Autodesk Fusion 360 part; units mm, degrees
(part 2 of 2)
  spline S15 degree 5 poles (15.988634, 0.602981) (15.980531, 0.608149) (15.964319, 0.618461) (15.939982, 0.633849) (15.907494, 0.654209) (15.866821, 0.679398) (15.826084, 0.704324) (15.785284, 0.728987) (15.744422, 0.753386) (15.703497, 0.777518) (15.662512, 0.801383) (15.621467, 0.824978) (15.580364, 0.848302) (15.539203, 0.871354) (15.497987, 0.89413) (15.456715, 0.916631) (15.415389, 0.938854) (15.37401, 0.960797) (15.332579, 0.98246) (15.291097, 1.003839) (15.249564, 1.024933) (15.207982, 1.04574) (15.166352, 1.066257) (15.124674, 1.086484) (15.082952, 1.106417) (15.041184, 1.126055) (14.999373, 1.145396) (14.957519, 1.164437) (14.915624, 1.183176) (14.873688, 1.201611) (14.831714, 1.219738) (14.789702, 1.237554) (14.747652, 1.255057) (14.705568, 1.272243) (14.663449, 1.28911) (14.621297, 1.305656) (14.579113, 1.321879) (14.536899, 1.337776) (14.494656, 1.353344) (14.452384, 1.368578) (14.410087, 1.383471) (14.367764, 1.398017) (14.325417, 1.412211) (14.283049, 1.426048) (14.24066, 1.439527) (14.198251, 1.452649) (14.155825, 1.465414) (14.113381, 1.47782) (14.070923, 1.48986) (14.028452, 1.501522) (13.98597, 1.512783) (13.94348, 1.523626) (13.900982, 1.534034) (13.858481, 1.544002) (13.815976, 1.553541) (13.773469, 1.562672) (13.73096, 1.571415) (13.688453, 1.579774) (13.64595, 1.587728) (13.603455, 1.595217) (13.560973, 1.60215) (13.518509, 1.608443) (13.476069, 1.614042) (13.433654, 1.618949) (13.391265, 1.62326) (13.348902, 1.627116) (13.306566, 1.630627) (13.264262, 1.633807) (13.222004, 1.636509) (13.179816, 1.638338) (13.137727, 1.638758) (13.104158, 1.637534) (13.079047, 1.635547) (13.062338, 1.633722) (13.053992, 1.632684) knots -1 -1 -1 -1 -1 -1 -0.98571429 -0.97142857 -0.95714286 -0.94285714 -0.92857143 -0.91428571 -0.9 -0.88571429 -0.87142857 -0.85714286 -0.84285714 -0.82857143 -0.81428571 -0.8 -0.78571429 -0.77142857 -0.75714286 -0.74285714 -0.72857143 -0.71428571 -0.7 -0.68571429 -0.67142857 -0.65714286 -0.64285714 -0.62857143 -0.61428571 -0.6 -0.58571429 -0.57142857 -0.55714286 -0.54285714 -0.52857143 -0.51428571 -0.5 -0.48571429 -0.47142857 -0.45714286 -0.44285714 -0.42857143 -0.41428571 -0.4 -0.38571429 -0.37142857 -0.35714286 -0.34285714 -0.32857143 -0.31428571 -0.3 -0.28571429 -0.27142857 -0.25714286 -0.24285714 -0.22857143 -0.21428571 -0.2 -0.18571429 -0.17142857 -0.15714286 -0.14285714 -0.12857143 -0.11428571 -0.1 -0.08571429 -0.07142857 -0.05714286 -0.04285714 -0.02857143 -0.01428571 0 0 0 0 0 0
  line L15 (13.053992, 1.632684) -> (12.411729, 1.552852)
  arc A31 (11.309164, 2.342397) -> (12.411729, 1.552852) centre (12.288381, 2.545216) ccw
  arc A32 (11.309164, 2.342397) -> (11.205533, 2.796436) centre (0, 0) ccw
  arc A33 (11.856339, 3.986176) -> (11.205533, 2.796436) centre (12.175776, 3.038568) ccw
  line L16 (11.856339, 3.986176) -> (12.469635, 4.192917)
  spline S16 degree 5 poles (12.469635, 4.192917) (12.477606, 4.195604) (12.493452, 4.201209) (12.516938, 4.210313) (12.547714, 4.223776) (12.585452, 4.242417) (12.622669, 4.262369) (12.659569, 4.283138) (12.696304, 4.304359) (12.732924, 4.325891) (12.769419, 4.347745) (12.80574, 4.370021) (12.841825, 4.392845) (12.877633, 4.416304) (12.913161, 4.440398) (12.948428, 4.465077) (12.983466, 4.490262) (13.018309, 4.51587) (13.052979, 4.541844) (13.087484, 4.568165) (13.12182, 4.594835) (13.155977, 4.621871) (13.189945, 4.649293) (13.223717, 4.67711) (13.257296, 4.705314) (13.290684, 4.733893) (13.32389, 4.762827) (13.356919, 4.792097) (13.389776, 4.82169) (13.422463, 4.851599) (13.454978, 4.881822) (13.487322, 4.912358) (13.519491, 4.943207) (13.551485, 4.974369) (13.583305, 5.005838) (13.614952, 5.037608) (13.646428, 5.069674) (13.677733, 5.102029) (13.708869, 5.134668) (13.739836, 5.167588) (13.770635, 5.200784) (13.801264, 5.234256) (13.831724, 5.268) (13.862015, 5.302013) (13.892137, 5.336294) (13.92209, 5.370838) (13.951874, 5.405642) (13.981489, 5.440703) (14.010937, 5.476018) (14.040216, 5.511585) (14.069326, 5.5474) (14.098269, 5.583462) (14.127042, 5.619769) (14.155647, 5.656317) (14.184084, 5.693105) (14.212351, 5.730131) (14.24045, 5.767391) (14.268379, 5.804885) (14.296139, 5.842609) (14.32373, 5.880561) (14.351152, 5.918741) (14.378404, 5.957145) (14.405487, 5.995773) (14.4324, 6.034621) (14.459143, 6.073689) (14.485715, 6.112973) (14.512116, 6.152472) (14.538345, 6.192183) (14.564404, 6.232106) (14.590291, 6.272239) (14.616007, 6.312581) (14.636444, 6.345021) (14.651694, 6.369445) (14.661827, 6.385769) (14.666885, 6.393941) knots 0 0 0 0 0 0 0.01428571 0.02857143 0.04285714 0.05714286 0.07142857 0.08571429 0.1 0.11428571 0.12857143 0.14285714 0.15714286 0.17142857 0.18571429 0.2 0.21428571 0.22857143 0.24285714 0.25714286 0.27142857 0.28571429 0.3 0.31428571 0.32857143 0.34285714 0.35714286 0.37142857 0.38571429 0.4 0.41428571 0.42857143 0.44285714 0.45714286 0.47142857 0.48571429 0.5 0.51428571 0.52857143 0.54285714 0.55714286 0.57142857 0.58571429 0.6 0.61428571 0.62857143 0.64285714 0.65714286 0.67142857 0.68571429 0.7 0.71428571 0.72857143 0.74285714 0.75714286 0.77142857 0.78571429 0.8 0.81428571 0.82857143 0.84285714 0.85714286 0.87142857 0.88571429 0.9 0.91428571 0.92857143 0.94285714 0.95714286 0.97142857 0.98571429 1 1 1 1 1 1
  arc A34 (14.666885, 6.393941) -> (14.143638, 7.480475) centre (0, 0) ccw
  spline S17 degree 5 poles (14.143638, 7.480475) (14.134095, 7.481616) (14.115014, 7.483872) (14.086411, 7.487177) (14.048306, 7.491425) (14.000732, 7.496472) (13.953214, 7.501255) (13.905754, 7.505773) (13.858352, 7.510026) (13.81101, 7.514012) (13.763729, 7.51773) (13.716511, 7.52118) (13.669358, 7.52436) (13.622272, 7.52727) (13.575255, 7.529908) (13.528308, 7.532273) (13.481432, 7.534365) (13.43463, 7.536182) (13.387903, 7.537722) (13.341253, 7.538986) (13.29468, 7.53997) (13.248189, 7.540675) (13.201779, 7.541098) (13.155453, 7.541238) (13.109213, 7.541095) (13.063062, 7.540666) (13.016999, 7.53995) (12.971029, 7.538946) (12.925152, 7.537652) (12.879371, 7.536066) (12.833688, 7.534185) (12.788106, 7.532009) (12.742627, 7.529533) (12.697253, 7.526758) (12.651987, 7.52368) (12.606831, 7.520298) (12.561786, 7.516612) (12.516854, 7.512619) (12.472039, 7.508317) (12.427345, 7.503701) (12.382774, 7.498767) (12.338331, 7.493509) (12.29402, 7.487924) (12.249843, 7.482008) (12.205804, 7.47576) (12.161902, 7.469182) (12.118138, 7.462274) (12.074515, 7.455036) (12.031038, 7.447463) (11.987713, 7.439541) (11.944552, 7.431256) (11.901565, 7.422589) (11.85876, 7.413527) (11.816142, 7.404067) (11.773708, 7.394219) (11.731448, 7.384003) (11.689356, 7.373437) (11.647432, 7.362524) (11.605687, 7.35125) (11.564151, 7.339558) (11.522868, 7.327373) (11.481879, 7.314618) (11.441212, 7.301249) (11.400868, 7.287267) (11.360807, 7.272759) (11.320966, 7.257852) (11.281299, 7.242646) (11.241805, 7.227157) (11.20256, 7.211256) (11.163756, 7.194599) (11.125653, 7.176716) (11.095939, 7.161048) (11.074177, 7.148363) (11.059915, 7.139469) (11.052845, 7.134912) knots -1 -1 -1 -1 -1 -1 -0.98571429 -0.97142857 -0.95714286 -0.94285714 -0.92857143 -0.91428571 -0.9 -0.88571429 -0.87142857 -0.85714286 -0.84285714 -0.82857143 -0.81428571 -0.8 -0.78571429 -0.77142857 -0.75714286 -0.74285714 -0.72857143 -0.71428571 -0.7 -0.68571429 -0.67142857 -0.65714286 -0.64285714 -0.62857143 -0.61428571 -0.6 -0.58571429 -0.57142857 -0.55714286 -0.54285714 -0.52857143 -0.51428571 -0.5 -0.48571429 -0.47142857 -0.45714286 -0.44285714 -0.42857143 -0.41428571 -0.4 -0.38571429 -0.37142857 -0.35714286 -0.34285714 -0.32857143 -0.31428571 -0.3 -0.28571429 -0.27142857 -0.25714286 -0.24285714 -0.22857143 -0.21428571 -0.2 -0.18571429 -0.17142857 -0.15714286 -0.14285714 -0.12857143 -0.11428571 -0.1 -0.08571429 -0.07142857 -0.05714286 -0.04285714 -0.02857143 -0.01428571 0 0 0 0 0 0
  line L17 (11.052845, 7.134912) -> (10.508824, 6.784319)
  arc A35 (9.172877, 7.017289) -> (10.508824, 6.784319) centre (9.967121, 7.624889) ccw
  arc A36 (9.172877, 7.017289) -> (8.882508, 7.3814) centre (0, 0) ccw
  arc A37 (8.952656, 8.735693) -> (8.882508, 7.3814) centre (9.65161, 8.020527) ccw
  line L18 (8.952656, 8.735693) -> (9.415515, 9.18806)
  spline S18 degree 5 poles (9.415515, 9.18806) (9.42153, 9.193938) (9.433375, 9.205864) (9.450585, 9.224257) (9.472472, 9.24974) (9.498385, 9.282909) (9.523259, 9.317033) (9.547494, 9.351755) (9.571383, 9.386813) (9.595034, 9.422102) (9.618433, 9.457627) (9.641492, 9.493455) (9.6641, 9.529676) (9.686184, 9.566348) (9.707739, 9.603471) (9.728806, 9.641008) (9.749447, 9.678901) (9.769728, 9.717091) (9.789696, 9.755536) (9.809364, 9.794221) (9.828727, 9.833148) (9.847771, 9.872327) (9.866477, 9.911771) (9.884836, 9.951486) (9.902851, 9.991467) (9.920534, 10.031702) (9.937897, 10.072178) (9.954955, 10.11288) (9.971719, 10.153799) (9.988191, 10.194928) (10.004374, 10.236266) (10.020265, 10.277811) (10.035863, 10.319563) (10.051168, 10.36152) (10.066183, 10.403679) (10.080912, 10.446035) (10.095357, 10.488582) (10.109524, 10.531315) (10.123415, 10.574232) (10.137032, 10.617327) (10.150377, 10.660599) (10.163451, 10.704046) (10.176254, 10.747664) (10.188787, 10.791452) (10.201052, 10.835407) (10.21305, 10.879526) (10.224784, 10.923806) (10.236254, 10.968245) (10.247462, 11.012839) (10.25841, 11.057587) (10.269098, 11.102487) (10.279528, 11.147535) (10.289699, 11.19273) (10.299614, 11.238071) (10.309272, 11.283554) (10.318675, 11.329178) (10.327825, 11.37494) (10.33672, 11.420838) (10.345364, 11.466871) (10.353755, 11.513036) (10.361896, 11.559333) (10.369786, 11.605758) (10.377427, 11.652311) (10.384819, 11.698989) (10.391963, 11.745791) (10.398858, 11.792714) (10.405507, 11.839756) (10.411909, 11.886916) (10.418065, 11.934192) (10.423976, 11.981582) (10.429642, 12.029087) (10.433979, 12.067181) (10.437122, 12.095803) (10.439169, 12.114907) (10.44018, 12.124465) knots 0 0 0 0 0 0 0.01428571 0.02857143 0.04285714 0.05714286 0.07142857 0.08571429 0.1 0.11428571 0.12857143 0.14285714 0.15714286 0.17142857 0.18571429 0.2 0.21428571 0.22857143 0.24285714 0.25714286 0.27142857 0.28571429 0.3 0.31428571 0.32857143 0.34285714 0.35714286 0.37142857 0.38571429 0.4 0.41428571 0.42857143 0.44285714 0.45714286 0.47142857 0.48571429 0.5 0.51428571 0.52857143 0.54285714 0.55714286 0.57142857 0.58571429 0.6 0.61428571 0.62857143 0.64285714 0.65714286 0.67142857 0.68571429 0.7 0.71428571 0.72857143 0.74285714 0.75714286 0.77142857 0.78571429 0.8 0.81428571 0.82857143 0.84285714 0.85714286 0.87142857 0.88571429 0.9 0.91428571 0.92857143 0.94285714 0.95714286 0.97142857 0.98571429 1 1 1 1 1 1
  arc A38 (10.44018, 12.124465) -> (9.497321, 12.87637) centre (0, 0) ccw
  spline S19 degree 5 poles (9.497321, 12.87637) (9.488228, 12.873257) (9.470058, 12.867011) (9.442853, 12.857578) (9.406679, 12.844872) (9.361626, 12.828778) (9.316739, 12.81247) (9.272018, 12.795948) (9.227466, 12.779213) (9.183082, 12.762263) (9.13887, 12.745099) (9.094832, 12.72772) (9.050969, 12.710127) (9.007283, 12.692318) (8.963777, 12.674295) (8.920453, 12.656057) (8.877312, 12.637603) (8.834357, 12.618933) (8.791589, 12.600047) (8.74901, 12.580944) (8.706623, 12.561624) (8.664429, 12.542087) (8.622432, 12.522332) (8.580633, 12.502358) (8.539035, 12.482166) (8.49764, 12.461755) (8.45645, 12.441124) (8.415467, 12.420274) (8.374695, 12.399203) (8.334136, 12.37791) (8.293793, 12.356395) (8.253669, 12.334657) (8.213768, 12.312694) (8.174092, 12.290506) (8.134644, 12.268093) (8.095427, 12.245454) (8.056442, 12.222588) (8.017693, 12.199495) (7.979183, 12.176175) (7.940917, 12.152624) (7.902901, 12.12884) (7.86514, 12.10482) (7.827641, 12.080562) (7.790406, 12.056064) (7.753439, 12.031327) (7.716738, 12.006351) (7.680306, 11.98114) (7.644143, 11.955691) (7.608257, 11.930004) (7.57266, 11.904069) (7.537368, 11.877877) (7.502399, 11.851416) (7.467765, 11.82468) (7.433472, 11.797666) (7.399512, 11.770382) (7.365871, 11.742842) (7.332532, 11.715058) (7.299494, 11.687037) (7.266775, 11.658766) (7.234425, 11.630211) (7.202517, 11.60132) (7.171121, 11.572044) (7.140282, 11.542354) (7.110001, 11.512252) (7.080201, 11.481799) (7.050774, 11.451082) (7.021633, 11.420171) (6.99277, 11.38908) (6.964311, 11.357726) (6.936577, 11.325882) (6.910006, 11.293238) (6.890033, 11.266229) (6.875931, 11.245358) (6.86694, 11.231156) (6.862547, 11.223984) knots -1 -1 -1 -1 -1 -1 -0.98571429 -0.97142857 -0.95714286 -0.94285714 -0.92857143 -0.91428571 -0.9 -0.88571429 -0.87142857 -0.85714286 -0.84285714 -0.82857143 -0.81428571 -0.8 -0.78571429 -0.77142857 -0.75714286 -0.74285714 -0.72857143 -0.71428571 -0.7 -0.68571429 -0.67142857 -0.65714286 -0.64285714 -0.62857143 -0.61428571 -0.6 -0.58571429 -0.57142857 -0.55714286 -0.54285714 -0.52857143 -0.51428571 -0.5 -0.48571429 -0.47142857 -0.45714286 -0.44285714 -0.42857143 -0.41428571 -0.4 -0.38571429 -0.37142857 -0.35714286 -0.34285714 -0.32857143 -0.31428571 -0.3 -0.28571429 -0.27142857 -0.25714286 -0.24285714 -0.22857143 -0.21428571 -0.2 -0.18571429 -0.17142857 -0.15714286 -0.14285714 -0.12857143 -0.11428571 -0.1 -0.08571429 -0.07142857 -0.05714286 -0.04285714 -0.02857143 -0.01428571 0 0 0 0 0 0
  line L19 (6.862547, 11.223984) -> (6.524518, 10.672068)
  arc A39 (5.219789, 10.302321) -> (6.524518, 10.672068) centre (5.67175, 11.194359) ccw
  arc A40 (5.219789, 10.302321) -> (4.800194, 10.504388) centre (0, 0) ccw
  arc A41 (4.275789, 11.754999) -> (4.800194, 10.504388) centre (5.215824, 11.413921) ccw
  line L20 (4.275789, 11.754999) -> (4.496536, 12.363394)
  spline S20 degree 5 poles (4.496536, 12.363394) (4.499405, 12.371301) (4.504902, 12.387185) (4.512427, 12.411223) (4.52109, 12.443679) (4.530046, 12.484806) (4.537651, 12.526344) (4.54442, 12.568143) (4.550733, 12.610094) (4.556731, 12.65215) (4.562399, 12.694309) (4.567628, 12.736594) (4.572282, 12.779037) (4.576267, 12.82166) (4.579581, 12.864459) (4.582275, 12.907419) (4.58443, 12.950515) (4.586133, 12.993723) (4.587443, 13.037024) (4.588378, 13.080412) (4.588935, 13.123885) (4.589093, 13.167447) (4.588832, 13.211101) (4.588141, 13.254849) (4.587026, 13.298687) (4.5855, 13.34261) (4.583582, 13.386611) (4.581291, 13.430684) (4.57864, 13.474823) (4.575636, 13.519027) (4.57228, 13.563292) (4.568571, 13.607618) (4.564509, 13.652003) (4.560094, 13.696446) (4.555331, 13.740944) (4.550223, 13.785496) (4.544778, 13.830097) (4.539, 13.874746) (4.532895, 13.919439) (4.526465, 13.964175) (4.519713, 14.008952) (4.512641, 14.053768) (4.505251, 14.098622) (4.497544, 14.143511) (4.489523, 14.188435) (4.481191, 14.23339) (4.47255, 14.278377) (4.463603, 14.323391) (4.454353, 14.368433) (4.444801, 14.413499) (4.434949, 14.45859) (4.4248, 14.503702) (4.414355, 14.548835) (4.403615, 14.593987) (4.392583, 14.639156) (4.381259, 14.684342) (4.369647, 14.729542) (4.357747, 14.774754) (4.345562, 14.819979) (4.333092, 14.865213) (4.320339, 14.910457) (4.307305, 14.955709) (4.293991, 15.000966) (4.280397, 15.046229) (4.266527, 15.091496) (4.252381, 15.136764) (4.23796, 15.182032) (4.223266, 15.227299) (4.208301, 15.272564) (4.193064, 15.317826) (4.177557, 15.363084) (4.164936, 15.399288) (4.15535, 15.42644) (4.148905, 15.44454) (4.145669, 15.45359) knots 0 0 0 0 0 0 0.01428571 0.02857143 0.04285714 0.05714286 0.07142857 0.08571429 0.1 0.11428571 0.12857143 0.14285714 0.15714286 0.17142857 0.18571429 0.2 0.21428571 0.22857143 0.24285714 0.25714286 0.27142857 0.28571429 0.3 0.31428571 0.32857143 0.34285714 0.35714286 0.37142857 0.38571429 0.4 0.41428571 0.42857143 0.44285714 0.45714286 0.47142857 0.48571429 0.5 0.51428571 0.52857143 0.54285714 0.55714286 0.57142857 0.58571429 0.6 0.61428571 0.62857143 0.64285714 0.65714286 0.67142857 0.68571429 0.7 0.71428571 0.72857143 0.74285714 0.75714286 0.77142857 0.78571429 0.8 0.81428571 0.82857143 0.84285714 0.85714286 0.87142857 0.88571429 0.9 0.91428571 0.92857143 0.94285714 0.95714286 0.97142857 0.98571429 1 1 1 1 1 1
  arc A42 (4.145669, 15.45359) -> (2.969943, 15.721941) centre (0, 0) ccw
  spline S21 degree 5 poles (2.969943, 15.721941) (2.963101, 15.715192) (2.949441, 15.70168) (2.929023, 15.681378) (2.901944, 15.654235) (2.868336, 15.620187) (2.834969, 15.586018) (2.801846, 15.551729) (2.768967, 15.51732) (2.736333, 15.482792) (2.703947, 15.448144) (2.671809, 15.413379) (2.639924, 15.378496) (2.608291, 15.343497) (2.576914, 15.308383) (2.545793, 15.273153) (2.514932, 15.237808) (2.484331, 15.202349) (2.453993, 15.166777) (2.423919, 15.131092) (2.394112, 15.095294) (2.364574, 15.059385) (2.335307, 15.023364) (2.306313, 14.987233) (2.277596, 14.950992) (2.249156, 14.914641) (2.220996, 14.878182) (2.193119, 14.841614) (2.165527, 14.80494) (2.138223, 14.768158) (2.11121, 14.731269) (2.084492, 14.694274) (2.058072, 14.657174) (2.031952, 14.619969) (2.006135, 14.58266) (1.980624, 14.545246) (1.955421, 14.50773) (1.930529, 14.470112) (1.905951, 14.432392) (1.881693, 14.39457) (1.857761, 14.356647) (1.834162, 14.318622) (1.810901, 14.280496) (1.787983, 14.242269) (1.76541, 14.203942) (1.74318, 14.165516) (1.721295, 14.126994) (1.699755, 14.088375) (1.678568, 14.049661) (1.657749, 14.01085) (1.637316, 13.971939) (1.617291, 13.932926) (1.597687, 13.893811) (1.578511, 13.854593) (1.559753, 13.815276) (1.541392, 13.775866) (1.52341, 13.736369) (1.505802, 13.696788) (1.488589, 13.657121) (1.471832, 13.617357) (1.45562, 13.577483) (1.440035, 13.537484) (1.425133, 13.497354) (1.41091, 13.457094) (1.397275, 13.416728) (1.38409, 13.376284) (1.371246, 13.335791) (1.358732, 13.295256) (1.346694, 13.254659) (1.335524, 13.213935) (1.325748, 13.172995) (1.319471, 13.139995) (1.315822, 13.115072) (1.313883, 13.098376) (1.313037, 13.090007) knots -1 -1 -1 -1 -1 -1 -0.98571429 -0.97142857 -0.95714286 -0.94285714 -0.92857143 -0.91428571 -0.9 -0.88571429 -0.87142857 -0.85714286 -0.84285714 -0.82857143 -0.81428571 -0.8 -0.78571429 -0.77142857 -0.75714286 -0.74285714 -0.72857143 -0.71428571 -0.7 -0.68571429 -0.67142857 -0.65714286 -0.64285714 -0.62857143 -0.61428571 -0.6 -0.58571429 -0.57142857 -0.55714286 -0.54285714 -0.52857143 -0.51428571 -0.5 -0.48571429 -0.47142857 -0.45714286 -0.44285714 -0.42857143 -0.41428571 -0.4 -0.38571429 -0.37142857 -0.35714286 -0.34285714 -0.32857143 -0.31428571 -0.3 -0.28571429 -0.27142857 -0.25714286 -0.24285714 -0.22857143 -0.21428571 -0.2 -0.18571429 -0.17142857 -0.15714286 -0.14285714 -0.12857143 -0.11428571 -0.1 -0.08571429 -0.07142857 -0.05714286 -0.04285714 -0.02857143 -0.01428571 0 0 0 0 0 0
  line L21 (1.313037, 13.090007) -> (1.24795, 12.446084)
  arc A43 (0.232858, 11.546852) -> (1.24795, 12.446084) centre (0.25302, 12.546649) ccw
  arc A44 (0.232858, 11.546852) -> (-0.232858, 11.546852) centre (0, 0) ccw
  arc A45 (-1.24795, 12.446084) -> (-0.232858, 11.546852) centre (-0.25302, 12.546649) ccw
  line L22 (-1.24795, 12.446084) -> (-1.313037, 13.090007)
  spline S22 degree 5 poles (-1.313037, 13.090007) (-1.313883, 13.098376) (-1.315822, 13.115072) (-1.319471, 13.139995) (-1.325748, 13.172995) (-1.335524, 13.213935) (-1.346694, 13.254659) (-1.358732, 13.295256) (-1.371246, 13.335791) (-1.38409, 13.376284) (-1.397275, 13.416728) (-1.41091, 13.457094) (-1.425133, 13.497354) (-1.440035, 13.537484) (-1.45562, 13.577483) (-1.471832, 13.617357) (-1.488589, 13.657121) (-1.505802, 13.696788) (-1.52341, 13.736369) (-1.541392, 13.775866) (-1.559753, 13.815276) (-1.578511, 13.854593) (-1.597687, 13.893811) (-1.617291, 13.932926) (-1.637316, 13.971939) (-1.657749, 14.01085) (-1.678568, 14.049661) (-1.699755, 14.088375) (-1.721295, 14.126994) (-1.74318, 14.165516) (-1.76541, 14.203942) (-1.787983, 14.242269) (-1.810901, 14.280496) (-1.834162, 14.318622) (-1.857761, 14.356647) (-1.881693, 14.39457) (-1.905951, 14.432392) (-1.930529, 14.470112) (-1.955421, 14.50773) (-1.980624, 14.545246) (-2.006135, 14.58266) (-2.031952, 14.619969) (-2.058072, 14.657174) (-2.084492, 14.694274) (-2.11121, 14.731269) (-2.138223, 14.768158) (-2.165527, 14.80494) (-2.193119, 14.841614) (-2.220996, 14.878182) (-2.249156, 14.914641) (-2.277596, 14.950992) (-2.306313, 14.987233) (-2.335307, 15.023364) (-2.364574, 15.059385) (-2.394112, 15.095294) (-2.423919, 15.131092) (-2.453993, 15.166777) (-2.484331, 15.202349) (-2.514932, 15.237808) (-2.545793, 15.273153) (-2.576914, 15.308383) (-2.608291, 15.343497) (-2.639924, 15.378496) (-2.671809, 15.413379) (-2.703947, 15.448144) (-2.736333, 15.482792) (-2.768967, 15.51732) (-2.801846, 15.551729) (-2.834969, 15.586018) (-2.868336, 15.620187) (-2.901944, 15.654235) (-2.929023, 15.681378) (-2.949441, 15.70168) (-2.963101, 15.715192) (-2.969943, 15.721941) knots 0 0 0 0 0 0 0.01428571 0.02857143 0.04285714 0.05714286 0.07142857 0.08571429 0.1 0.11428571 0.12857143 0.14285714 0.15714286 0.17142857 0.18571429 0.2 0.21428571 0.22857143 0.24285714 0.25714286 0.27142857 0.28571429 0.3 0.31428571 0.32857143 0.34285714 0.35714286 0.37142857 0.38571429 0.4 0.41428571 0.42857143 0.44285714 0.45714286 0.47142857 0.48571429 0.5 0.51428571 0.52857143 0.54285714 0.55714286 0.57142857 0.58571429 0.6 0.61428571 0.62857143 0.64285714 0.65714286 0.67142857 0.68571429 0.7 0.71428571 0.72857143 0.74285714 0.75714286 0.77142857 0.78571429 0.8 0.81428571 0.82857143 0.84285714 0.85714286 0.87142857 0.88571429 0.9 0.91428571 0.92857143 0.94285714 0.95714286 0.97142857 0.98571429 1 1 1 1 1 1
  arc A46 (-2.969943, 15.721941) -> (-4.145669, 15.45359) centre (0, 0) ccw
  spline S23 degree 5 poles (-4.145669, 15.45359) (-4.148905, 15.44454) (-4.15535, 15.42644) (-4.164936, 15.399288) (-4.177557, 15.363084) (-4.193064, 15.317826) (-4.208301, 15.272564) (-4.223266, 15.227299) (-4.23796, 15.182032) (-4.252381, 15.136764) (-4.266527, 15.091496) (-4.280397, 15.046229) (-4.293991, 15.000966) (-4.307305, 14.955709) (-4.320339, 14.910457) (-4.333092, 14.865213) (-4.345562, 14.819979) (-4.357747, 14.774754) (-4.369647, 14.729542) (-4.381259, 14.684342) (-4.392583, 14.639156) (-4.403615, 14.593987) (-4.414355, 14.548835) (-4.4248, 14.503702) (-4.434949, 14.45859) (-4.444801, 14.413499) (-4.454353, 14.368433) (-4.463603, 14.323391) (-4.47255, 14.278377) (-4.481191, 14.23339) (-4.489523, 14.188435) (-4.497544, 14.143511) (-4.505251, 14.098622) (-4.512641, 14.053768) (-4.519713, 14.008952) (-4.526465, 13.964175) (-4.532895, 13.919439) (-4.539, 13.874746) (-4.544778, 13.830097) (-4.550223, 13.785496) (-4.555331, 13.740944) (-4.560094, 13.696446) (-4.564509, 13.652003) (-4.568571, 13.607618) (-4.57228, 13.563292) (-4.575636, 13.519027) (-4.57864, 13.474823) (-4.581291, 13.430684) (-4.583582, 13.386611) (-4.5855, 13.34261) (-4.587026, 13.298687) (-4.588141, 13.254849) (-4.588832, 13.211101) (-4.589093, 13.167447) (-4.588935, 13.123885) (-4.588378, 13.080412) (-4.587443, 13.037024) (-4.586133, 12.993723) (-4.58443, 12.950515) (-4.582275, 12.907419) (-4.579581, 12.864459) (-4.576267, 12.82166) (-4.572282, 12.779037) (-4.567628, 12.736594) (-4.562399, 12.694309) (-4.556731, 12.65215) (-4.550733, 12.610094) (-4.54442, 12.568143) (-4.537651, 12.526344) (-4.530046, 12.484806) (-4.52109, 12.443679) (-4.512427, 12.411223) (-4.504902, 12.387185) (-4.499405, 12.371301) (-4.496536, 12.363394) knots -1 -1 -1 -1 -1 -1 -0.98571429 -0.97142857 -0.95714286 -0.94285714 -0.92857143 -0.91428571 -0.9 -0.88571429 -0.87142857 -0.85714286 -0.84285714 -0.82857143 -0.81428571 -0.8 -0.78571429 -0.77142857 -0.75714286 -0.74285714 -0.72857143 -0.71428571 -0.7 -0.68571429 -0.67142857 -0.65714286 -0.64285714 -0.62857143 -0.61428571 -0.6 -0.58571429 -0.57142857 -0.55714286 -0.54285714 -0.52857143 -0.51428571 -0.5 -0.48571429 -0.47142857 -0.45714286 -0.44285714 -0.42857143 -0.41428571 -0.4 -0.38571429 -0.37142857 -0.35714286 -0.34285714 -0.32857143 -0.31428571 -0.3 -0.28571429 -0.27142857 -0.25714286 -0.24285714 -0.22857143 -0.21428571 -0.2 -0.18571429 -0.17142857 -0.15714286 -0.14285714 -0.12857143 -0.11428571 -0.1 -0.08571429 -0.07142857 -0.05714286 -0.04285714 -0.02857143 -0.01428571 0 0 0 0 0 0
  line L23 (-4.496536, 12.363394) -> (-4.275789, 11.754999)
  arc A47 (-4.800194, 10.504388) -> (-4.275789, 11.754999) centre (-5.215824, 11.413921) ccw
  arc A48 (-4.800194, 10.504388) -> (-5.219789, 10.302321) centre (0, 0) ccw
  arc A49 (-6.524518, 10.672068) -> (-5.219789, 10.302321) centre (-5.67175, 11.194359) ccw
  line L24 (-6.524518, 10.672068) -> (-6.862547, 11.223984)
  spline S24 degree 5 poles (-6.862547, 11.223984) (-6.86694, 11.231156) (-6.875931, 11.245358) (-6.890033, 11.266229) (-6.910006, 11.293238) (-6.936577, 11.325882) (-6.964311, 11.357726) (-6.99277, 11.38908) (-7.021633, 11.420171) (-7.050774, 11.451082) (-7.080201, 11.481799) (-7.110001, 11.512252) (-7.140282, 11.542354) (-7.171121, 11.572044) (-7.202517, 11.60132) (-7.234425, 11.630211) (-7.266775, 11.658766) (-7.299494, 11.687037) (-7.332532, 11.715058) (-7.365871, 11.742842) (-7.399512, 11.770382) (-7.433472, 11.797666) (-7.467765, 11.82468) (-7.502399, 11.851416) (-7.537368, 11.877877) (-7.57266, 11.904069) (-7.608257, 11.930004) (-7.644143, 11.955691) (-7.680306, 11.98114) (-7.716738, 12.006351) (-7.753439, 12.031327) (-7.790406, 12.056064) (-7.827641, 12.080562) (-7.86514, 12.10482) (-7.902901, 12.12884) (-7.940917, 12.152624) (-7.979183, 12.176175) (-8.017693, 12.199495) (-8.056442, 12.222588) (-8.095427, 12.245454) (-8.134644, 12.268093) (-8.174092, 12.290506) (-8.213768, 12.312694) (-8.253669, 12.334657) (-8.293793, 12.356395) (-8.334136, 12.37791) (-8.374695, 12.399203) (-8.415467, 12.420274) (-8.45645, 12.441124) (-8.49764, 12.461755) (-8.539035, 12.482166) (-8.580633, 12.502358) (-8.622432, 12.522332) (-8.664429, 12.542087) (-8.706623, 12.561624) (-8.74901, 12.580944) (-8.791589, 12.600047) (-8.834357, 12.618933) (-8.877312, 12.637603) (-8.920453, 12.656057) (-8.963777, 12.674295) (-9.007283, 12.692318) (-9.050969, 12.710127) (-9.094832, 12.72772) (-9.13887, 12.745099) (-9.183082, 12.762263) (-9.227466, 12.779213) (-9.272018, 12.795948) (-9.316739, 12.81247) (-9.361626, 12.828778) (-9.406679, 12.844872) (-9.442853, 12.857578) (-9.470058, 12.867011) (-9.488228, 12.873257) (-9.497321, 12.87637) knots 0 0 0 0 0 0 0.01428571 0.02857143 0.04285714 0.05714286 0.07142857 0.08571429 0.1 0.11428571 0.12857143 0.14285714 0.15714286 0.17142857 0.18571429 0.2 0.21428571 0.22857143 0.24285714 0.25714286 0.27142857 0.28571429 0.3 0.31428571 0.32857143 0.34285714 0.35714286 0.37142857 0.38571429 0.4 0.41428571 0.42857143 0.44285714 0.45714286 0.47142857 0.48571429 0.5 0.51428571 0.52857143 0.54285714 0.55714286 0.57142857 0.58571429 0.6 0.61428571 0.62857143 0.64285714 0.65714286 0.67142857 0.68571429 0.7 0.71428571 0.72857143 0.74285714 0.75714286 0.77142857 0.78571429 0.8 0.81428571 0.82857143 0.84285714 0.85714286 0.87142857 0.88571429 0.9 0.91428571 0.92857143 0.94285714 0.95714286 0.97142857 0.98571429 1 1 1 1 1 1
  arc A50 (-9.497321, 12.87637) -> (-10.44018, 12.124465) centre (0, 0) ccw
  spline S25 degree 5 poles (-10.44018, 12.124465) (-10.439169, 12.114907) (-10.437122, 12.095803) (-10.433979, 12.067181) (-10.429642, 12.029087) (-10.423976, 11.981582) (-10.418065, 11.934192) (-10.411909, 11.886916) (-10.405507, 11.839756) (-10.398858, 11.792714) (-10.391963, 11.745791) (-10.384819, 11.698989) (-10.377427, 11.652311) (-10.369786, 11.605758) (-10.361896, 11.559333) (-10.353755, 11.513036) (-10.345364, 11.466871) (-10.33672, 11.420838) (-10.327825, 11.37494) (-10.318675, 11.329178) (-10.309272, 11.283554) (-10.299614, 11.238071) (-10.289699, 11.19273) (-10.279528, 11.147535) (-10.269098, 11.102487) (-10.25841, 11.057587) (-10.247462, 11.012839) (-10.236254, 10.968245) (-10.224784, 10.923806) (-10.21305, 10.879526) (-10.201052, 10.835407) (-10.188787, 10.791452) (-10.176254, 10.747664) (-10.163451, 10.704046) (-10.150377, 10.660599) (-10.137032, 10.617327) (-10.123415, 10.574232) (-10.109524, 10.531315) (-10.095357, 10.488582) (-10.080912, 10.446035) (-10.066183, 10.403679) (-10.051168, 10.36152) (-10.035863, 10.319563) (-10.020265, 10.277811) (-10.004374, 10.236266) (-9.988191, 10.194928) (-9.971719, 10.153799) (-9.954955, 10.11288) (-9.937897, 10.072178) (-9.920534, 10.031702) (-9.902851, 9.991467) (-9.884836, 9.951486) (-9.866477, 9.911771) (-9.847771, 9.872327) (-9.828727, 9.833148) (-9.809364, 9.794221) (-9.789696, 9.755536) (-9.769728, 9.717091) (-9.749447, 9.678901) (-9.728806, 9.641008) (-9.707739, 9.603471) (-9.686184, 9.566348) (-9.6641, 9.529676) (-9.641492, 9.493455) (-9.618433, 9.457627) (-9.595034, 9.422102) (-9.571383, 9.386813) (-9.547494, 9.351755) (-9.523259, 9.317033) (-9.498385, 9.282909) (-9.472472, 9.24974) (-9.450585, 9.224257) (-9.433375, 9.205864) (-9.42153, 9.193938) (-9.415515, 9.18806) knots -1 -1 -1 -1 -1 -1 -0.98571429 -0.97142857 -0.95714286 -0.94285714 -0.92857143 -0.91428571 -0.9 -0.88571429 -0.87142857 -0.85714286 -0.84285714 -0.82857143 -0.81428571 -0.8 -0.78571429 -0.77142857 -0.75714286 -0.74285714 -0.72857143 -0.71428571 -0.7 -0.68571429 -0.67142857 -0.65714286 -0.64285714 -0.62857143 -0.61428571 -0.6 -0.58571429 -0.57142857 -0.55714286 -0.54285714 -0.52857143 -0.51428571 -0.5 -0.48571429 -0.47142857 -0.45714286 -0.44285714 -0.42857143 -0.41428571 -0.4 -0.38571429 -0.37142857 -0.35714286 -0.34285714 -0.32857143 -0.31428571 -0.3 -0.28571429 -0.27142857 -0.25714286 -0.24285714 -0.22857143 -0.21428571 -0.2 -0.18571429 -0.17142857 -0.15714286 -0.14285714 -0.12857143 -0.11428571 -0.1 -0.08571429 -0.07142857 -0.05714286 -0.04285714 -0.02857143 -0.01428571 0 0 0 0 0 0
  line L25 (-9.415515, 9.18806) -> (-8.952656, 8.735693)
  arc A51 (-8.882508, 7.3814) -> (-8.952656, 8.735693) centre (-9.65161, 8.020527) ccw
  arc A52 (-8.882508, 7.3814) -> (-9.172877, 7.017289) centre (0, 0) ccw
  arc A53 (-10.508824, 6.784319) -> (-9.172877, 7.017289) centre (-9.967121, 7.624889) ccw
  line L26 (-10.508824, 6.784319) -> (-11.052845, 7.134912)
  spline S26 degree 5 poles (-11.052845, 7.134912) (-11.059915, 7.139469) (-11.074177, 7.148363) (-11.095939, 7.161048) (-11.125653, 7.176716) (-11.163756, 7.194599) (-11.20256, 7.211256) (-11.241805, 7.227157) (-11.281299, 7.242646) (-11.320966, 7.257852) (-11.360807, 7.272759) (-11.400868, 7.287267) (-11.441212, 7.301249) (-11.481879, 7.314618) (-11.522868, 7.327373) (-11.564151, 7.339558) (-11.605687, 7.35125) (-11.647432, 7.362524) (-11.689356, 7.373437) (-11.731448, 7.384003) (-11.773708, 7.394219) (-11.816142, 7.404067) (-11.85876, 7.413527) (-11.901565, 7.422589) (-11.944552, 7.431256) (-11.987713, 7.439541) (-12.031038, 7.447463) (-12.074515, 7.455036) (-12.118138, 7.462274) (-12.161902, 7.469182) (-12.205804, 7.47576) (-12.249843, 7.482008) (-12.29402, 7.487924) (-12.338331, 7.493509) (-12.382774, 7.498767) (-12.427345, 7.503701) (-12.472039, 7.508317) (-12.516854, 7.512619) (-12.561786, 7.516612) (-12.606831, 7.520298) (-12.651987, 7.52368) (-12.697253, 7.526758) (-12.742627, 7.529533) (-12.788106, 7.532009) (-12.833688, 7.534185) (-12.879371, 7.536066) (-12.925152, 7.537652) (-12.971029, 7.538946) (-13.016999, 7.53995) (-13.063062, 7.540666) (-13.109213, 7.541095) (-13.155453, 7.541238) (-13.201779, 7.541098) (-13.248189, 7.540675) (-13.29468, 7.53997) (-13.341253, 7.538986) (-13.387903, 7.537722) (-13.43463, 7.536182) (-13.481432, 7.534365) (-13.528308, 7.532273) (-13.575255, 7.529908) (-13.622272, 7.52727) (-13.669358, 7.52436) (-13.716511, 7.52118) (-13.763729, 7.51773) (-13.81101, 7.514012) (-13.858352, 7.510026) (-13.905754, 7.505773) (-13.953214, 7.501255) (-14.000732, 7.496472) (-14.048306, 7.491425) (-14.086411, 7.487177) (-14.115014, 7.483872) (-14.134095, 7.481616) (-14.143638, 7.480475) knots 0 0 0 0 0 0 0.01428571 0.02857143 0.04285714 0.05714286 0.07142857 0.08571429 0.1 0.11428571 0.12857143 0.14285714 0.15714286 0.17142857 0.18571429 0.2 0.21428571 0.22857143 0.24285714 0.25714286 0.27142857 0.28571429 0.3 0.31428571 0.32857143 0.34285714 0.35714286 0.37142857 0.38571429 0.4 0.41428571 0.42857143 0.44285714 0.45714286 0.47142857 0.48571429 0.5 0.51428571 0.52857143 0.54285714 0.55714286 0.57142857 0.58571429 0.6 0.61428571 0.62857143 0.64285714 0.65714286 0.67142857 0.68571429 0.7 0.71428571 0.72857143 0.74285714 0.75714286 0.77142857 0.78571429 0.8 0.81428571 0.82857143 0.84285714 0.85714286 0.87142857 0.88571429 0.9 0.91428571 0.92857143 0.94285714 0.95714286 0.97142857 0.98571429 1 1 1 1 1 1
  arc A54 (-14.143638, 7.480475) -> (-14.666885, 6.393941) centre (0, 0) ccw
  spline S27 degree 5 poles (-14.666885, 6.393941) (-14.661827, 6.385769) (-14.651694, 6.369445) (-14.636444, 6.345021) (-14.616007, 6.312581) (-14.590291, 6.272239) (-14.564404, 6.232106) (-14.538345, 6.192183) (-14.512116, 6.152472) (-14.485715, 6.112973) (-14.459143, 6.073689) (-14.4324, 6.034621) (-14.405487, 5.995773) (-14.378404, 5.957145) (-14.351152, 5.918741) (-14.32373, 5.880561) (-14.296139, 5.842609) (-14.268379, 5.804885) (-14.24045, 5.767391) (-14.212351, 5.730131) (-14.184084, 5.693105) (-14.155647, 5.656317) (-14.127042, 5.619769) (-14.098269, 5.583462) (-14.069326, 5.5474) (-14.040216, 5.511585) (-14.010937, 5.476018) (-13.981489, 5.440703) (-13.951874, 5.405642) (-13.92209, 5.370838) (-13.892137, 5.336294) (-13.862015, 5.302013) (-13.831724, 5.268) (-13.801264, 5.234256) (-13.770635, 5.200784) (-13.739836, 5.167588) (-13.708869, 5.134668) (-13.677733, 5.102029) (-13.646428, 5.069674) (-13.614952, 5.037608) (-13.583305, 5.005838) (-13.551485, 4.974369) (-13.519491, 4.943207) (-13.487322, 4.912358) (-13.454978, 4.881822) (-13.422463, 4.851599) (-13.389776, 4.82169) (-13.356919, 4.792097) (-13.32389, 4.762827) (-13.290684, 4.733893) (-13.257296, 4.705314) (-13.223717, 4.67711) (-13.189945, 4.649293) (-13.155977, 4.621871) (-13.12182, 4.594835) (-13.087484, 4.568165) (-13.052979, 4.541844) (-13.018309, 4.51587) (-12.983466, 4.490262) (-12.948428, 4.465077) (-12.913161, 4.440398) (-12.877633, 4.416304) (-12.841825, 4.392845) (-12.80574, 4.370021) (-12.769419, 4.347745) (-12.732924, 4.325891) (-12.696304, 4.304359) (-12.659569, 4.283138) (-12.622669, 4.262369) (-12.585452, 4.242417) (-12.547714, 4.223776) (-12.516938, 4.210313) (-12.493452, 4.201209) (-12.477606, 4.195604) (-12.469635, 4.192917) knots -1 -1 -1 -1 -1 -1 -0.98571429 -0.97142857 -0.95714286 -0.94285714 -0.92857143 -0.91428571 -0.9 -0.88571429 -0.87142857 -0.85714286 -0.84285714 -0.82857143 -0.81428571 -0.8 -0.78571429 -0.77142857 -0.75714286 -0.74285714 -0.72857143 -0.71428571 -0.7 -0.68571429 -0.67142857 -0.65714286 -0.64285714 -0.62857143 -0.61428571 -0.6 -0.58571429 -0.57142857 -0.55714286 -0.54285714 -0.52857143 -0.51428571 -0.5 -0.48571429 -0.47142857 -0.45714286 -0.44285714 -0.42857143 -0.41428571 -0.4 -0.38571429 -0.37142857 -0.35714286 -0.34285714 -0.32857143 -0.31428571 -0.3 -0.28571429 -0.27142857 -0.25714286 -0.24285714 -0.22857143 -0.21428571 -0.2 -0.18571429 -0.17142857 -0.15714286 -0.14285714 -0.12857143 -0.11428571 -0.1 -0.08571429 -0.07142857 -0.05714286 -0.04285714 -0.02857143 -0.01428571 0 0 0 0 0 0
  line L27 (-12.469635, 4.192917) -> (-11.856339, 3.986176)
  arc A55 (-11.205533, 2.796436) -> (-11.856339, 3.986176) centre (-12.175776, 3.038568) ccw
  circle A56 centre (0, 0) radius 1.5
  line L28 (1.118034, -1) -> (-1.118034, -1)
  circle A57 centre (0, 0) radius 1.6
  line L29 (1.118034, -1.1) -> (-1.118034, -1.1)
  line L30 (1.118034, -1.1) -> (1.161897, -1.099998)
  line L31 (-1.118034, -1.1) -> (-1.161895, -1.1)
  point P0 (0, 1.5)
  dimension "d9" = 3
  dimension "d10" = 2.5
  dimension "d13" = 0.1
  dimension "d14" = -0.1
  constraint coincident A0.centre A2.centre
  constraint horizontal L28
  constraint coincident A56 P0
  constraint parallel L29 L30
  constraint parallel L29 L31
  measures "d9" diameter of A56
  measures "d10" distance of L28 P0
extrude "Transfer_Gear (4)" cut sketch "Transfer_Gear" against normal blind 8 contours A56 L28 | A56 A57 L29 L30 L31 | A56 L28 L29 picked at (0.367719, -0.32787) picked at (1.336694, -0.745781) picked at (-0.362112, -1.011449) in component "Transfer_Gear"
sketch "Transfer_Gear (2)" plane through (0, 0, 0) normal (0, 1, 0) x (1, 0, 0)
  line L0 (15.988634, 0) -> (15.988634, -9)
  line L1 (8.952656, 0) -> (8.65161, 0)
  line L2 (8.952656, 0) -> (9.415515, 0)
  line L3 (9.415515, 0) -> (10.44018, 0)
  line L4 (9.497321, 0) -> (10.44018, 0)
  line L5 (6.862547, 0) -> (9.497321, 0)
  line L6 (6.862547, 0) -> (6.524518, 0)
  line L7 (6.524518, 0) -> (5.219789, 0)
  line L8 (4.800194, 0) -> (5.219789, 0)
  line L9 (4.800194, 0) -> (4.215824, 0)
  line L10 (4.275789, 0) -> (4.496536, 0)
  line L11 (4.588992, 0) -> (4.145669, 0)
  line L12 (2.969943, 0) -> (4.145669, 0)
  line L13 (1.313037, 0) -> (2.969943, 0)
  line L14 (1.313037, 0) -> (1.24795, 0)
  line L15 (1.24795, 0) -> (0.232858, 0)
  line L16 (-0.232858, 0) -> (0.232858, 0)
  line L17 (-0.232858, 0) -> (-1.24795, 0)
  line L18 (-1.24795, 0) -> (-1.313037, 0)
  line L19 (-1.313037, 0) -> (-2.969943, 0)
  line L20 (-4.145669, 0) -> (-2.969943, 0)
  line L21 (-4.588992, 0) -> (-4.145669, 0)
  line L22 (-4.496536, 0) -> (-4.275789, 0)
  line L23 (-4.215824, 0) -> (-4.800194, 0)
  line L24 (-5.219789, 0) -> (-4.800194, 0)
  line L25 (-5.219789, 0) -> (-6.524518, 0)
  line L26 (-6.524518, 0) -> (-6.862547, 0)
  line L27 (-6.862547, 0) -> (-9.497321, 0)
  line L28 (-10.44018, 0) -> (-9.497321, 0)
  line L29 (-9.415515, 0) -> (-10.44018, 0)
  line L30 (-9.415515, 0) -> (-8.952656, 0)
  line L31 (-8.65161, 0) -> (-8.952656, 0)
  line L32 (-9.172877, 0) -> (-8.882508, 0)
  line L33 (-9.172877, 0) -> (-10.508824, 0)
  line L34 (-10.508824, 0) -> (-11.052845, 0)
  line L35 (-11.052845, 0) -> (-14.143638, 0)
  line L36 (-14.666885, 0) -> (-14.143638, 0)
  line L37 (-12.469635, 0) -> (-14.666885, 0)
  line L38 (-12.469635, 0) -> (-11.856339, 0)
  line L39 (-11.175776, 0) -> (-11.856339, 0)
  line L40 (-11.309164, 0) -> (-11.205533, 0)
  line L41 (-11.309164, 0) -> (-12.411729, 0)
  line L42 (-12.411729, 0) -> (-13.053992, 0)
  line L43 (-13.053992, 0) -> (-15.988634, 0)
  line L44 (-16, 0) -> (-15.988634, 0)
  line L45 (-13.053992, 0) -> (-15.988634, 0)
  line L46 (-13.053992, 0) -> (-12.411729, 0)
  line L47 (-11.309164, 0) -> (-12.411729, 0)
  line L48 (-11.309164, 0) -> (-11.205533, 0)
  line L49 (-11.175776, 0) -> (-11.856339, 0)
  line L50 (-11.856339, 0) -> (-12.469635, 0)
  line L51 (-12.469635, 0) -> (-14.666885, 0)
  line L52 (-14.666885, 0) -> (-14.143638, 0)
  line L53 (-11.052845, 0) -> (-14.143638, 0)
  line L54 (-11.052845, 0) -> (-10.508824, 0)
  line L55 (-9.172877, 0) -> (-10.508824, 0)
  line L56 (-9.172877, 0) -> (-8.882508, 0)
  line L57 (-8.65161, 0) -> (-8.952656, 0)
  line L58 (-8.952656, 0) -> (-9.415515, 0)
  line L59 (-9.415515, 0) -> (-10.44018, 0)
  line L60 (-10.44018, 0) -> (-9.497321, 0)
  line L61 (-6.862547, 0) -> (-9.497321, 0)
  line L62 (-6.862547, 0) -> (-6.524518, 0)
  line L63 (-5.219789, 0) -> (-6.524518, 0)
  line L64 (-5.219789, 0) -> (-4.800194, 0)
  line L65 (-4.215824, 0) -> (-4.800194, 0)
  line L66 (-4.275789, 0) -> (-4.496536, 0)
  line L67 (-4.588992, 0) -> (-4.145669, 0)
  line L68 (-4.145669, 0) -> (-2.969943, 0)
  line L69 (-1.313037, 0) -> (-2.969943, 0)
  line L70 (-1.313037, 0) -> (-1.24795, 0)
  line L71 (-0.232858, 0) -> (-1.24795, 0)
  line L72 (-0.232858, 0) -> (0.232858, 0)
  line L73 (1.24795, 0) -> (0.232858, 0)
  line L74 (1.24795, 0) -> (1.313037, 0)
  line L75 (1.313037, 0) -> (2.969943, 0)
  line L76 (2.969943, 0) -> (4.145669, 0)
  line L77 (4.588992, 0) -> (4.145669, 0)
  line L78 (4.496536, 0) -> (4.275789, 0)
  line L79 (4.800194, 0) -> (4.215824, 0)
  line L80 (4.800194, 0) -> (5.219789, 0)
  line L81 (6.524518, 0) -> (5.219789, 0)
  line L82 (6.524518, 0) -> (6.862547, 0)
  line L83 (6.862547, 0) -> (9.497321, 0)
  line L84 (9.497321, 0) -> (10.44018, 0)
  line L85 (9.415515, 0) -> (10.44018, 0)
  line L86 (9.415515, 0) -> (8.952656, 0)
  line L87 (8.952656, 0) -> (8.65161, 0)
  line L88 (8.882508, 0) -> (9.172877, 0)
  line L89 (10.508824, 0) -> (9.172877, 0)
  line L90 (10.508824, 0) -> (11.052845, 0)
  line L91 (11.052845, 0) -> (14.143638, 0)
  line L92 (14.143638, 0) -> (14.666885, 0)
  line L93 (12.469635, 0) -> (14.666885, 0)
  line L94 (12.469635, 0) -> (11.856339, 0)
  line L95 (11.856339, 0) -> (11.175776, 0)
  line L96 (11.205533, 0) -> (11.309164, 0)
  line L97 (12.411729, 0) -> (11.309164, 0)
  line L98 (12.411729, 0) -> (13.053992, 0)
  line L99 (13.053992, 0) -> (15.988634, 0)
  line L100 (15.988634, 0) -> (16, 0)
  line L101 (13.053992, 0) -> (15.988634, 0)
  line L102 (13.053992, 0) -> (12.411729, 0)
  line L103 (12.411729, 0) -> (11.309164, 0)
  line L104 (11.205533, 0) -> (11.309164, 0)
  line L105 (11.856339, 0) -> (11.175776, 0)
  line L106 (11.856339, 0) -> (12.469635, 0)
  line L107 (12.469635, 0) -> (14.666885, 0)
  line L108 (14.143638, 0) -> (14.666885, 0)
  line L109 (11.052845, 0) -> (14.143638, 0)
  line L110 (11.052845, 0) -> (10.508824, 0)
  line L111 (10.508824, 0) -> (9.172877, 0)
  line L112 (8.882508, 0) -> (9.172877, 0)
  line L113 (6.524518, 0) -> (15.988634, -5.157552)
  line L114 (15.988634, -5.157552) -> (17.5, -5.157552)
  line L115 (17.5, -5.157552) -> (17.5, 1.5)
  line L116 (17.5, 1.5) -> (6.524518, 1.5)
  line L117 (6.524518, 1.5) -> (6.524518, 0)
  constraint perpendicular L0 L114
  constraint perpendicular L114 L115
  constraint perpendicular L115 L116
  constraint perpendicular L82 L117
revolve "Transfer_Gear (5)" cut sketch "Transfer_Gear (2)" angle 360 about axis through (0, 0, 1.75) along (0, 0, 1) contours L0 L1 L2 L3 L4 L5 L6 L82 L83 L84 L85 L86 L87 L88 L89 L90 L91 L92 L93 L94 L95 L96 L97 L98 L99 L101 L102 L103 L104 L105 L106 L107 L108 L109 L110 L111 L112 L114 L115 L116 L117 | L0 L1 L2 L3 L4 L5 L6 L82 L83 L84 L85 L86 L87 L88 L89 L90 L91 L92 L93 L94 L95 L96 L97 L98 L99 L101 L102 L103 L104 L105 L106 L107 L108 L109 L110 L111 L112 L113 picked at (11.511114, 1) picked at (15.548051, -1.719184) in component "Transfer_Gear"
fillet "Transfer_Gear (6)" radius 0.4 2 faces at (-2.076837, 7.769014, 9) (1.472282, -1.92845, 0) in component "Transfer_Gear"
component "Transfer_Gear" placed x (1, 0, 0) y (0, 1, 0) z (0, 0, 1) at (0, 0, 0)
